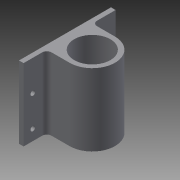
# Autodesk Inventor part: Motor_Mount_3DPrint
Saved by Autodesk Inventor 2015 SP1 (Build 190203100, 203)
## iProperties
Created: 2016-04-07
Part Number: Motor_Mount_3DPrint
Material: Generic
Document SubType Name: Modeling
Designer: Ethan
Density: 1 g/cm^3
Appearance: Default
Author: Ethan
Autodesk Inventor part; units mm, degrees
ref_plane "YZ Plane" through (0, 0, 0) normal (1, 0, 0) x (0, 1, 0)
ref_plane "XZ Plane" through (0, 0, 0) normal (0, 1, 0) x (-1, 0, 0)
ref_plane "XY Plane" through (0, 0, 0) normal (0, 0, 1) x (1, 0, 0)
sketch "Sketch1" plane through (0, 0, 0) normal (0, 1, 0) x (-1, 0, 0)
  line L0 (0, 31.75) -> (-3.175, 31.75)
  line L1 (-3.175, -31.75) -> (0, -31.75)
  line L2 (0, -31.75) -> (0, 31.75)
  circle A0 centre (-18.85, 0) radius 12.5
  circle A1 centre (-18.85, 0) radius 12.2
  arc A2 (-18.85, 15.675) -> (-18.85, -15.675) centre (-18.85, 0) ccw
  line L3 (-18.85, 15.675) -> (-6.35, 15.675)
  line L4 (-18.85, -15.675) -> (-6.35, -15.675)
  line L5 (-3.175, 31.75) -> (-3.175, 18.85)
  line L6 (-3.175, -18.85) -> (-3.175, -31.75)
  arc A3 (-6.35, 15.675) -> (-3.175, 18.85) centre (-6.35, 18.85) ccw
  arc A4 (-3.175, -18.85) -> (-6.35, -15.675) centre (-6.35, -18.85) ccw
  point P0 (0, 0)
  dimension "d0" = 3.175
  dimension "d1" = 63.5
  dimension "d4" = 25
  dimension "d6" = 24.4
  dimension "d7" = 31.35
  dimension "d8" = 3.175
  dimension "d26" = 3.175
  dimension "d27" = 18.85
  constraints: 14 end point, 6 point on circle, 5 centre point, 5 tangent, 4 parallel, 4 perpendicular, 2 coincident, 1 equal radius, 1 horizontal
  measures "d0" distance of L0.start L0.end
  measures "d1" distance of L1.end L0.start
  measures "d4" diameter of A0
  measures "d6" diameter of A1
  measures "d7" diameter of A2
  measures "d8" radius of A3
  measures "d26" distance of L1.start L1.end
  measures "d27" distance from line of L2 A0.centre
extrude "Extrusion1" add sketch "Sketch1" along normal blind 49.8 contours L2 L1 L6 A4 L4 A2 L3 A3 L5 L0
extrude "Extrusion2" add sketch "Sketch1" along normal blind 30.8 contours A0
sketch "Sketch2" plane through (3.175, 0, 31.75) normal (1, 0, 0) x (0, 0, -1)
  line L0 (63.5, 0) -> (63.5, 49.8) projected
  line L1 (0, 0) -> (0, 49.8) projected
  circle A0 centre (6.35, 28.6333) radius 1.5875
  circle A1 centre (6.35, 7.4667) radius 1.5875
  line L2 (0, 49.8) -> (12.9, 49.8) projected
  line L3 (31.75, 0) -> (31.75, 49.8)
  line L4 (19.25, 49.8) -> (44.25, 49.8) projected
  circle A2 centre (57.15, 28.6333) radius 1.5875
  circle A3 centre (57.15, 7.4667) radius 1.5875
  dimension "d14" = 63.5
  dimension "d16" = 3.175
  dimension "d17" = 3.175
  dimension "d18" = 21.1667
  dimension "d19" = 21.1667
  dimension "d20" = 0
  dimension "d21" = 6.35
  dimension "d22" = 31.75
  constraints: 4 centre point, 2 end point, 2 symmetric about line, 1 midpoint, 2 other
  measures "d14" distance between parallel lines of L0 L1
  measures "d16" diameter of A0
  measures "d17" diameter of A1
  measures "d18" distance of A0.centre A1.centre
  measures "d19" distance from line of L2 A0.centre
  measures "d20" horizontal distance of A1.centre A0.centre
  measures "d21" distance from line of L1 A0.centre
  measures "d22" distance between parallel lines of L3 L1
extrude "Extrusion3" cut sketch "Sketch2" against normal blind 3.175
body "Solid1"
